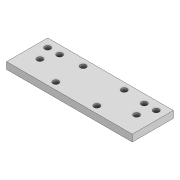
# Autodesk Inventor part: drag chain mount
Saved by Autodesk Inventor 2020 (Build 240168000, 168)
## iProperties
Created: 2020-02-07
Part Number: drag chain mount
Material: Generic
Document SubType Name: Modeling
Designer: ball
Density: 1 g/cm^3
Appearance: Default
Author: ball
Autodesk Inventor part; units mm, degrees
ref_plane "YZ Plane" through (0, 0, 0) normal (1, 0, 0) x (0, 1, 0)
ref_plane "XZ Plane" through (0, 0, 0) normal (0, 1, 0) x (-1, 0, 0)
ref_plane "XY Plane" through (0, 0, 0) normal (0, 0, 1) x (1, 0, 0)
sketch "Sketch1" plane through (0, 0, 0) normal (0, 1, 0) x (-1, 0, 0)
  line L0 (0, 0) -> (35.5, 0)
  line L1 (35.5, 0) -> (35.5, -24)
  line L2 (35.5, -24) -> (0, -24)
  line L3 (0, -24) -> (0, 0)
  circle A0 centre (5.75, -20) radius 1.7
  circle A1 centre (5.75, -4) radius 1.7
  circle A2 centre (29.75, -20) radius 1.7
  circle A3 centre (29.75, -4) radius 1.7
  line L4 (0, -24) -> (-19, -24)
  line L5 (-19, -24) -> (-19, 0)
  line L6 (-19, 0) -> (0, 0)
  line L7 (0, 0) -> (0, -24)
  circle A4 centre (-14, -19) radius 1.7
  circle A5 centre (-7, -19) radius 1.7
  circle A6 centre (-10.5, -11) radius 1.7
  line L8 (35.5, 0) -> (54.5, 0)
  line L9 (54.5, 0) -> (54.5, -24)
  line L10 (54.5, -24) -> (35.5, -24)
  line L11 (35.5, -24) -> (35.5, 0)
  circle A7 centre (49.5, -19) radius 1.7
  circle A8 centre (46, -11) radius 1.7
  circle A9 centre (42.5, -19) radius 1.7
  dimension "d0" = 35.5
  dimension "d1" = 24
  dimension "d2" = 3.4
  dimension "d3" = 4
  dimension "d4" = 5.75
  dimension "d5" = 3.4
  dimension "d6" = 16
  dimension "d7" = 3.4
  dimension "d8" = 4
  dimension "d9" = 5.75
  dimension "d10" = 3.4
  dimension "d11" = 16
  dimension "d12" = 19
  dimension "d13" = 24
  dimension "d14" = 3.4
  dimension "d15" = 5
  dimension "d16" = 5
  dimension "d17" = 3.4
  dimension "d18" = 7
  dimension "d19" = 3.4
  dimension "d20" = 8
  dimension "d21" = 3.5
  dimension "d22" = 19
  dimension "d23" = 24
  dimension "d24" = 3.4
  dimension "d25" = 3.4
  dimension "d26" = 5
  dimension "d27" = 5
  dimension "d28" = 8
  dimension "d29" = 3.5
  dimension "d30" = 3.4
  dimension "d31" = 7
  dimension "d32" = 5
  constraints: 24 end point, 10 centre point, 6 parallel, 3 horizontal, 3 perpendicular
  measures "d0" distance of L1.end L2.end
  measures "d1" distance of L0.end L1.end
  measures "d2" diameter of A0
  measures "d3" distance from line of L2 A0.centre
  measures "d4" distance from line of L3 A0.centre
  measures "d5" diameter of A1
  measures "d6" distance of A0.centre A1.centre
  measures "d7" diameter of A2
  measures "d8" distance from line of L2 A2.centre
  measures "d9" distance from line of L1 A2.centre
  measures "d10" diameter of A3
  measures "d11" distance of A2.centre A3.centre
  measures "d12" distance of L5.end L6.end
  measures "d13" distance of L4.end L5.end
  measures "d14" diameter of A4
  measures "d15" distance from line of L5 A4.centre
  measures "d16" distance from line of L4 A4.centre
  measures "d17" diameter of A5
  measures "d18" distance of A4.centre A5.centre
  measures "d19" diameter of A6
  measures "d20" vertical distance of A4.centre A6.centre
  measures "d21" horizontal distance of A4.centre A6.centre
  measures "d22" distance of L9.end L10.end
  measures "d23" distance of L8.end L9.end
  measures "d24" diameter of A7
  measures "d25" diameter of A8
  measures "d26" distance from line of L10 A7.centre
  measures "d27" distance from line of L9 A7.centre
  measures "d28" vertical distance of A8.centre A7.centre
  measures "d29" horizontal distance of A8.centre A7.centre
  measures "d30" diameter of A9
  measures "d31" distance of A9.centre A7.centre
  measures "d32" distance from line of L10 A9.centre
extrude "Extrusion1" add sketch "Sketch1" along normal blind 4
body "Solid1"
